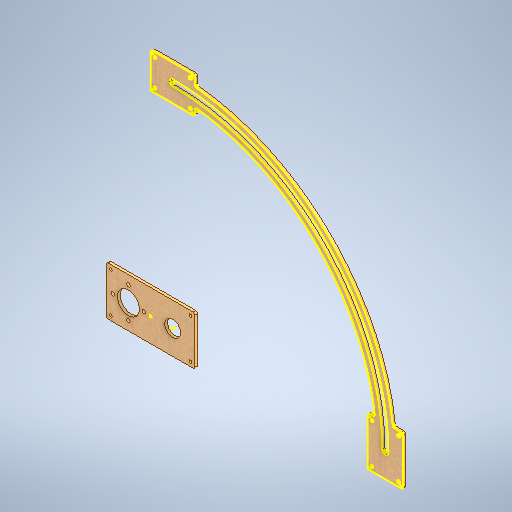
# Autodesk Inventor part: xx_plate_guide
Saved by Autodesk Inventor 2025.1 (Build 291241000, 241)
## iProperties
Created: 2024-12-04
Part Number: xx_plate_guide
Material: 一般
Document SubType Name: Modeling
Designer: yuki0520
Density: 1 g/cm^3
Appearance: イエロー パイン材 - 硬質 塗装 抑えた光沢
Author: yuki0520
Autodesk Inventor part; units mm, degrees
ref_plane "YZ Plane" through (0, 0, 0) normal (1, 0, 0) x (0, 1, 0)
ref_plane "XZ Plane" through (0, 0, 0) normal (0, 1, 0) x (-1, 0, 0)
ref_plane "XY Plane" through (0, 0, 0) normal (0, 0, 1) x (1, 0, 0)
sketch "スケッチ1" plane through (0, 0, 0) normal (0, 0, 1) x (1, 0, 0)
  line L0 (50, -27.5) -> (-50, -27.5)
  line L1 (-50, -27.5) -> (-50, 27.5)
  line L2 (-50, 27.5) -> (50, 27.5)
  line L3 (50, 27.5) -> (50, -27.5)
  line L4 (50, -27.5) -> (-50, 27.5) construction
  line L5 (-50, -27.5) -> (50, 27.5) construction
  circle A0 centre (0, 0) radius 25
  line L6 (-50, 0) -> (50, 0)
  circle A1 centre (25, 0) radius 9
  circle A2 centre (-25, 0) radius 12.5
  circle A3 centre (-25, 0) radius 17.5
  circle A4 centre (-25, 17.5) radius 2.05
  circle A5 centre (-42.5, 0) radius 2.05
  circle A6 centre (-25, -17.5) radius 2.05
  circle A7 centre (-7.5, 0) radius 2.05
  line L7 (0, 0) -> (240, 0) construction
  line L8 (0, 0) -> (240, 0) construction
  circle A8 centre (25, 0) radius 240
  circle A9 centre (25, 0) radius 230
  circle A10 centre (25, 0) radius 250
  circle A11 centre (25, 0) radius 236.5
  circle A12 centre (25, 0) radius 243.5
  line L9 (25, 0) -> (425, 0)
  line L10 (425, 0) -> (425, 400)
  line L11 (425, 400) -> (25, 400)
  line L12 (25, 400) -> (25, 0)
  line L13 (445, -27.5) -> (405, -27.5)
  line L14 (405, -27.5) -> (405, 27.5)
  line L15 (405, 27.5) -> (445, 27.5)
  line L16 (445, 27.5) -> (445, -27.5)
  line L17 (445, -27.5) -> (405, 27.5) construction
  line L18 (405, -27.5) -> (445, 27.5) construction
  line L19 (50, 220) -> (0, 220)
  line L20 (0, 220) -> (0, 260)
  line L21 (0, 260) -> (50, 260)
  line L22 (50, 260) -> (50, 220)
  line L23 (50, 220) -> (0, 260) construction
  line L24 (0, 220) -> (50, 260) construction
  line L25 (285, -27.5) -> (245, -27.5)
  line L26 (245, -27.5) -> (245, 27.5)
  line L27 (245, 27.5) -> (285, 27.5)
  line L28 (285, 27.5) -> (285, -27.5)
  line L29 (285, -27.5) -> (245, 27.5) construction
  line L30 (245, -27.5) -> (285, 27.5) construction
  circle A13 centre (25, 240) radius 3.5
  circle A14 centre (265, 0) radius 3.5
  point P0 (273.4829, 27.5)
  point P1 (25, 250)
  point P2 (25, 243.5)
  point P3 (266.9421, 27.5)
  point P4 (259.8957, 27.5)
  point P5 (25, 236.5)
  point P6 (25, 230)
  point P7 (253.3501, 27.5)
  point P8 (50, 248.7469)
  point P9 (50, 228.6373)
  point P10 (263.4193, -27.5)
  point P11 (261.5, 0)
  point P12 (266.9421, -27.5)
  point P13 (425, 27.5)
  point P14 (405, 0)
  point P15 (25, 220)
  point P16 (0, 228.6373)
  point P17 (255, 0)
  point P18 (0, 235.1749)
  point P19 (25, 240)
  point P20 (0, 238.6944)
  point P21 (0, 242.2132)
  point P22 (0, 248.7469)
  point P23 (25, 260)
  point P24 (275, 0)
  point P25 (268.5, 0)
  point P26 (50, 235.1749)
  point P27 (50, 238.6944)
  point P28 (50, 242.2132)
  point P29 (253.3501, 27.5)
  point P30 (273.4829, 27.5)
  point P31 (25, 236.5)
  point P32 (25, 243.5)
  point P33 (268.5, 0)
  point P34 (261.5, 0)
  dimension "d5" = 35
  dimension "d0" = 100
  dimension "d1" = 55
  dimension "d2" = 50
  dimension "d3" = 18
  dimension "d4" = 25
  dimension "d6" = 4.1
  dimension "d9" = 360
  dimension "d11" = 25
  dimension "d26" = 480
  dimension "d27" = 10
  dimension "d28" = 10
  dimension "d29" = 3.5
  dimension "d30" = 3.5
  dimension "d31" = 400
  dimension "d32" = 400
  dimension "d33" = 40
  dimension "d34" = 55
  dimension "d35" = 50
  dimension "d36" = 40
  dimension "d37" = 40
  dimension "d38" = 55
  constraints: 62 end point, 14 centre point, 11 midpoint, 10 parallel, 6 horizontal, 5 perpendicular, 5 point on circle, 4 coincident, 3 point on line, 2 tangent, 1 collinear, 1 vertical alignment, 11 other
  measures "d0" distance of L1.end L2.end
  measures "d1" distance of L0.end L1.end
  measures "d2" diameter of A0
  measures "d3" diameter of A1
  measures "d4" diameter of A2
  measures "d6" diameter of A4
  measures "d11" distance from line of L1 A4.centre
  measures "d26" diameter of A8
  measures "d27" radial gap between concentric circles of A8 A9
  measures "d28" radial gap between concentric circles of A8 A10
  measures "d29" radial gap between concentric circles of A8 A11
  measures "d30" radial gap between concentric circles of A8 A12
  measures "d31" distance of L11.end L10.end
  measures "d32" distance of L10.end L9.end
  measures "d33" distance of L14.end L15.end
  measures "d34" distance of L13.end L14.end
  measures "d35" distance of L20.end L21.end
  measures "d36" distance of L19.end L20.end
  measures "d37" distance of L26.end L27.end
  measures "d38" distance of L25.end L26.end
extrude "押し出し1" add sketch "スケッチ1" along normal blind 3 contours L0 L1 L6 A5 A3 A6 A0 A1 L3 | L6 A1 L12 L2 L3 | L1 L2 L12 A1 A0 A3 A4 A5 L6 | L26 L27 A9 L9 | L9 A9 L25 L26 | A0 A3 A7 L6 A1 | L9 A11 L25 A9 | A9 L27 A11 L9 | A3 A4 A0 A2 L6 A5 | A5 L6 A2 A0 A3 A6 | L19 L20 A9 L12 | L12 A9 L22 L19 | A1 L6 A7 A3 A0 | A0 A2 L6 A7 A3 | A9 L22 A11 L27 | A14 A8 L25 A11 | L12 A11 L22 A9 | A9 L20 A11 L12 | A3 A7 L6 A2 A0 | A14 A12 L25 A8 | A11 L20 A8 A13 | L9 A10 L25 A12 | A12 L27 A10 L9 | A8 L20 A12 A13 | A12 L22 A10 L27 | L9 L28 L25 A10 | A10 L27 L28 L9 | L12 A10 L22 A12 | A12 L20 A10 L12 | L12 L21 L22 A10 | A10 L20 L21 L12
sketch "スケッチ2" plane through (0, 0, 3) normal (0, 0, 1) x (1, 0, 0)
  line L0 (50, 27.5) -> (-50, 27.5) projected
  line L1 (-50, 27.5) -> (-50, -27.5) projected
  line L2 (-50, -27.5) -> (50, -27.5) projected
  line L3 (50, -27.5) -> (50, 27.5) projected
  circle A0 centre (25, 0) radius 9 projected
  circle A1 centre (-7.5, 0) radius 2.05 projected
  circle A2 centre (-25, 17.5) radius 2.05 projected
  circle A3 centre (-42.5, 0) radius 2.05 projected
  circle A4 centre (-25, -17.5) radius 2.05 projected
  circle A5 centre (-25, 0) radius 12.5 projected
  line L4 (-45, 22.5) -> (45, 22.5)
  line L5 (45, 22.5) -> (45, -22.5)
  line L6 (45, -22.5) -> (-45, -22.5)
  line L7 (-45, -22.5) -> (-45, 22.5)
  line L8 (0, 260) -> (0, 220) projected
  line L9 (0, 220) -> (50, 220) projected
  line L10 (50, 220) -> (50, 228.6373) projected
  arc A6 (253.3501, 27.5) -> (50, 228.6373) centre (25, 0) ccw projected
  line L11 (253.3501, 27.5) -> (245, 27.5) projected
  line L12 (245, 27.5) -> (245, -27.5) projected
  line L13 (245, -27.5) -> (285, -27.5) projected
  line L14 (285, -27.5) -> (285, 27.5) projected
  line L15 (285, 27.5) -> (273.4829, 27.5) projected
  arc A7 (273.4829, 27.5) -> (50, 248.7469) centre (25, 0) ccw projected
  line L16 (50, 248.7469) -> (50, 260) projected
  line L17 (50, 260) -> (0, 260) projected
  arc A8 (268.5, 0) -> (25, 243.5) centre (25, 0) ccw projected
  arc A9 (261.5, 0) -> (25, 236.5) centre (25, 0) ccw projected
  line L18 (280, -22.5) -> (250, -22.5)
  line L19 (250, -22.5) -> (250, 22.5)
  line L20 (250, 22.5) -> (258.9204, 22.5)
  arc A10 (258.9204, 22.5) -> (45, 234.1474) centre (25, 0) ccw
  line L21 (45, 234.1474) -> (45, 225)
  line L22 (45, 225) -> (5, 225)
  line L23 (5, 225) -> (5, 255)
  line L24 (5, 255) -> (45, 255)
  line L25 (45, 255) -> (45, 244.1823)
  arc A11 (268.9646, 22.5) -> (45, 244.1823) centre (25, 0) ccw
  line L26 (268.9646, 22.5) -> (280, 22.5)
  line L27 (280, 22.5) -> (280, -22.5)
  arc A12 (261.5, 0) -> (268.5, 0) centre (265, 0) ccw projected
  arc A13 (25, 243.5) -> (25, 236.5) centre (25, 240) ccw projected
  point P0 (0, 0)
  dimension "d14" = 5
  dimension "d39" = 5
  constraints: 28 end point, 12 coincident, 4 point on circle, 2 centre point, 14 other
  measures "d14" distance between parallel lines of L0 L4
  measures "d39" distance between parallel lines of L13 L18
hole "穴1" at (-45, 22.5, 3) at (-45, -22.5, 3) at (45, -22.5, 3) at (45, 22.5, 3) at (5, 225, 3) at (5, 255, 3) at (45, 255, 3) at (45, 225, 3) at (250, -22.5, 3) at (280, -22.5, 3) at (280, 22.5, 3) at (250, 22.5, 3) direction (0, 0, -1) diameter 3.2 end through all
fillet "フィレット1" radius 2 16 edges at (-50, 27.5, 1.5) (50, 27.5, 1.5) (50, -27.5, 1.5) (-50, -27.5, 1.5) (285, -27.5, 1.5) (285, 27.5, 1.5) (245, -27.5, 1.5) (245, 27.5, 1.5) (50, 260, 1.5) (50, 248.7469, 1.5) (0, 260, 1.5) (0, 220, 1.5) (50, 220, 1.5) (50, 228.6373, 1.5) (273.4829, 27.5, 1.5) (253.3501, 27.5, 1.5)
sketch "スケッチ3" plane through (0, 0, 3) normal (0, 0, 1) x (1, 0, 0)
  arc A0 (48, 220) -> (50, 222) centre (48, 222) ccw projected
  line L0 (50, 222) -> (50, 226.3957) projected
  arc A1 (52.2368, 228.3816) -> (50, 226.3957) centre (52, 226.3957) ccw projected
  arc A2 (253.0667, 29.7588) -> (52.2368, 228.3816) centre (25, 0) ccw projected
  arc A3 (251.0835, 27.5) -> (253.0667, 29.7588) centre (251.0835, 29.5) ccw projected
  line L1 (251.0835, 27.5) -> (247, 27.5) projected
  arc A4 (247, 27.5) -> (245, 25.5) centre (247, 25.5) ccw projected
  line L2 (245, 25.5) -> (245, -25.5) projected
  arc A5 (245, -25.5) -> (247, -27.5) centre (247, -25.5) ccw projected
  line L3 (247, -27.5) -> (283, -27.5) projected
  arc A6 (283, -27.5) -> (285, -25.5) centre (283, -25.5) ccw projected
  line L4 (285, -25.5) -> (285, 25.5) projected
  arc A7 (285, 25.5) -> (283, 27.5) centre (283, 25.5) ccw projected
  line L5 (283, 27.5) -> (275.2674, 27.5) projected
  arc A8 (273.2811, 29.2659) -> (275.2674, 27.5) centre (275.2674, 29.5) ccw projected
  arc A9 (273.2811, 29.2659) -> (51.7857, 248.5609) centre (25, 0) ccw projected
  arc A10 (50, 250.5494) -> (51.7857, 248.5609) centre (52, 250.5494) ccw projected
  line L6 (50, 250.5494) -> (50, 258) projected
  arc A11 (50, 258) -> (48, 260) centre (48, 258) ccw projected
  line L7 (48, 260) -> (2, 260) projected
  arc A12 (2, 260) -> (0, 258) centre (2, 258) ccw projected
  line L8 (0, 258) -> (0, 222) projected
  arc A13 (0, 222) -> (2, 220) centre (2, 222) ccw projected
  line L9 (2, 220) -> (48, 220) projected
  circle A14 centre (250, 22.5) radius 1.6 projected
  circle A15 centre (280, 22.5) radius 1.6 projected
  circle A16 centre (280, -22.5) radius 1.6 projected
  circle A17 centre (250, -22.5) radius 1.6 projected
  circle A18 centre (45, 225) radius 1.6 projected
  circle A19 centre (45, 255) radius 1.6 projected
  circle A20 centre (5, 255) radius 1.6 projected
  circle A21 centre (5, 225) radius 1.6 projected
  arc A22 (268.5, 0) -> (25, 243.5) centre (25, 0) ccw projected
  arc A23 (261.5, 0) -> (268.5, 0) centre (265, 0) ccw projected
  arc A24 (261.5, 0) -> (25, 236.5) centre (25, 0) ccw projected
  arc A25 (25, 243.5) -> (25, 236.5) centre (25, 240) ccw projected
  point P0 (0, 0)
equation "\"d11\" = -0.5 * d2 + 0.5 * d0"
equation "\"d34\" = d1"
equation "\"d36\" = d37"
equation "\"d38\" = d1"
